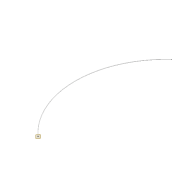
# Autodesk Inventor part: Landing_legs
Saved by Autodesk Inventor 2022 (Build 260153000, 153)
## iProperties
Created: 2022-04-29
Part Number: Landing_legs
Material: Generic
Document SubType Name: Modeling
Designer: dell
Density: 1 g/cm^3
Appearance: Default
Author: dell
Autodesk Inventor part; units mm, degrees
ref_plane "YZ Plane" through (0, 0, 0) normal (1, 0, 0) x (0, 1, 0)
ref_plane "XZ Plane" through (0, 0, 0) normal (0, 1, 0) x (-1, 0, 0)
ref_plane "XY Plane" through (0, 0, 0) normal (0, 0, 1) x (1, 0, 0)
sketch "Sketch1" plane through (0, 0, 0) normal (0, 1, 0) x (-1, 0, 0)
  line L0 (0, -1065.6) -> (0, 177.6) projected
  arc A0 (0, -888) -> (0, 0) centre (-403.5641, -444) ccw
  dimension "d4" = 888
  dimension "d5" = 600
  constraints: 2 point on circle, 1 centre point, 1 point on line
  measures "d4" distance of A0.end A0.start
  measures "d5" radius of A0
ref_plane "Work Plane1" through (0, 0, 0) normal (0.74, 0, 0.6726069) x (0, 1, 0)
sketch "Sketch2" plane through (0, 0, 0) normal (0.74, 0, 0.6726069) x (0, 1, 0)
  circle A0 centre (0, 0) radius 2
  dimension "d6" = 4
  constraints: 1 centre point, 1 coincident
  measures "d6" diameter of A0
sweep "Sweep1" add profiles "Sketch2" path "Sketch1" path curves A0
body "Solid1"
